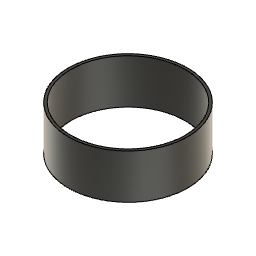
Layer v2 (Autodesk Fusion 360 design; units mm, degrees)
Autodesk Fusion 360 part; units mm, degrees
sketch "Sketch3" plane through (0, 0, 0) normal (0, 0, 1) x (1, 0, 0)
  circle A0 centre (0, 0) radius 45
  dimension "d43" = 90
  constraint coincident A0.centre origin
  measures "d43" diameter of A0
extrude "Extrude3" add sketch "Sketch3" along normal blind 35 thin wall 2 outside makes body 1
copy_body "Body->Comp3" bodies 1 removing the originals makes body 2 in component "Layer"
component "Layer" placed x (1, 0, 0) y (0, 1, 0) z (0, 0, 1) at (0, 0, 0)
equation "Diameter = 150 mm"
equation "Thickness = 35 mm"
equation "WaveAmplitude = 5 mm"
equation "WaveLength = 5"
equation "d43 = Diameter * 3 / 5"
equation "d45 = Thickness"
